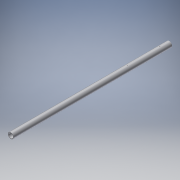
# Autodesk Inventor part: 2f2barm
Saved by Autodesk Inventor 2016 (Build 200138000, 138)
## iProperties
Company: HERA Project
Created: 2013-07-11
Part Number: 2f2barm
Material: PVC-Piping
Description: PVC arm for feed backplane
Document SubType Name: Modeling
Designer: David DeBoer
Mass: 174.937 g
Surface Area: 877.469 cm^2
Volume: 124.955 cm^3
Density: 1.4 g/cm^3
Appearance: Smooth - White
Title: feed-bppvcarm
Author: David DeBoer
Autodesk Inventor part; units mm, degrees
ref_plane "YZ Plane" through (0, 0, 0) normal (1, 0, 0) x (0, 1, 0)
ref_plane "XZ Plane" through (0, 0, 0) normal (0, 1, 0) x (-1, 0, 0)
ref_plane "XY Plane" through (0, 0, 0) normal (0, 0, 1) x (1, 0, 0)
sketch "Sketch1" plane through (0, 0, 0) normal (0, 0, 1) x (1, 0, 0)
  circle A0 centre (0, 0) radius 13.335
  circle A1 centre (0, 0) radius 10.4648
  dimension "d0" = 26.67
  dimension "d2" = 2.8702
  constraints: 2 centre point, 1 coincident
  measures "d0" diameter of A0
  measures "d2" radial gap between concentric circles of A1 A0
extrude "Extrusion1" add sketch "Sketch1" along normal blind 731.2
sketch "Sketch6" plane through (0, 0, 731.2) normal (0, 0, 1) x (1, 0, 0)
  circle A0 centre (0, 0) radius 10.4648 projected
  circle A1 centre (0, 0) radius 13.335 projected
  line L0 (-4.066, 12.7) -> (4.066, 12.7)
  dimension "d18" = 12.7
  constraints: 2 end point, 2 point on circle, 1 horizontal
  measures "d18" distance from line of A0.centre L0
extrude "Extrusion3" cut sketch "Sketch6" against normal through all contours L0 A1 picked at (-0.4583, 12.888)
sketch "Sketch7" plane through (-4.066, 12.7, 731.2) normal (0, 1, 0) x (1, 0, 0)
  circle A0 centre (4.066, 838.2) radius 1.27
  line L0 (0, 0) -> (0, 731.2) projected
  circle A1 centre (4.066, 688.2) radius 1.27
  circle A2 centre (4.066, 538.2) radius 1.27
  line L1 (8.132, 0) -> (0, 0) projected
  point P0 (4.066, 731.2)
  dimension "d23" = 2.54
  dimension "d34" = 150
  dimension "d46" = 838.2
  constraints: 3 centre point, 1 vertical, 4 other
  measures "d23" diameter of A0
  measures "d34" distance of A0.centre A1.centre
  measures "d46" distance from line of L1 A0.centre
hole "Hole3" at (0, 12.7, -107) at (0, 12.7, 43) at (0, 12.7, 193) direction (0, -1, 0) diameter 3.175 end through all
body "Solid1"
